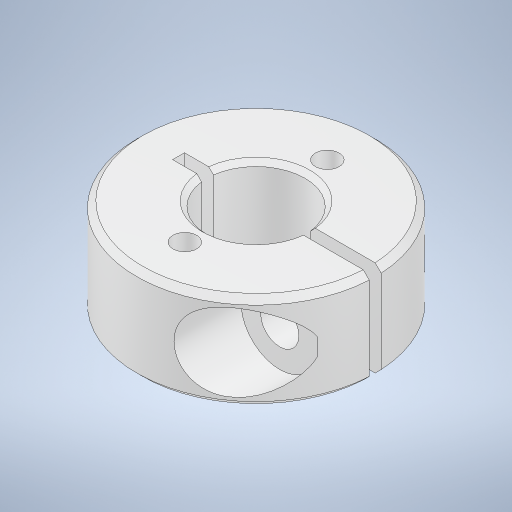
# Autodesk Inventor part: Collar
Saved by Autodesk Inventor 2023.4 (Build 274418000, 418)
## iProperties
Created: 2024-03-24
Part Number: Collar
Material: Aluminum 6061
Document SubType Name: Modeling
Designer: Nathan Cai
Density: 2.7 g/cm^3
Appearance: Aluminum - Flat
Author: Nathan Cai
Autodesk Inventor part; units mm, degrees
ref_plane "YZ Plane" through (0, 0, 0) normal (1, 0, 0) x (0, 1, 0)
ref_plane "XZ Plane" through (0, 0, 0) normal (0, 1, 0) x (-1, 0, 0)
sketch "Sketch1" plane through (0, 0, 0) normal (0, 1, 0) x (-1, 0, 0)
  circle A0 centre (0, 0) radius 4
  circle A1 centre (0, 0) radius 10
  dimension "d0" = 8
  dimension "d1" = 20
  constraints: 2 centre point, 2 coincident
  measures "d0" diameter of A0
  measures "d1" diameter of A1
extrude "Extrusion1" add sketch "Sketch1" along normal blind 8
chamfer "Chamfer1" distance 0.5 angle 45 4 edges at (4, 8, 0) (10, 8, 0) (10, 0, 0) (4, 0, 0)
thicken "Thicken1" operation add thickness 0.1 both sides no extend neighbours yes toward (-0.9967573, 0, -0.0804666) faces at (-3.987, 5.1667, -0.3219)
sketch "Sketch2" plane through (0, 8, 0) normal (0, 1, 0) x (1, 0, 0)
  circle A0 centre (0, 0) radius 4 construction
  line L0 (-4, 0) -> (0, 0) construction
  line L1 (9.9875, -0.5) -> (-6.5, -0.5)
  line L2 (-6.5, -0.5) -> (-6.5, 0.5)
  line L3 (-6.5, 0.5) -> (9.9875, 0.5)
  line L4 (9.9875, 0.5) -> (9.9875, -0.5) construction
  line L5 (9.9875, -0.5) -> (-6.5, 0.5) construction
  line L6 (-6.5, -0.5) -> (9.9875, 0.5) construction
  circle A1 centre (0, 0) radius 10 projected
  point P0 (1.7437, 0)
  dimension "d4" = 1
  dimension "d5" = 2.5
  constraints: 14 end point, 2 horizontal, 2 midpoint, 2 parallel, 1 horizontal alignment, 1 perpendicular, 1 point on line, 3 other
  measures "d4" distance of L1.end L2.end
  measures "d5" distance from line of L2 L0.start
extrude "Extrusion2" cut sketch "Sketch2" against normal through all contours L1 L2 L3 A1 picked at (-1, 0)
sketch "Sketch3" plane through (0, 0, 0) normal (0, -1, 0) x (1, 0, 0)
  circle A0 centre (0, 5.975) radius 1.875 construction
  arc A1 (4.0694, 0.5) -> (-4.0694, 0.5) centre (0, 0) ccw projected
  arc A2 (9.9875, 0.5) -> (9.9875, -0.5) centre (0, 0) ccw projected
  circle A3 centre (0, 5.975) radius 1
  line L0 (0, 0) -> (0, 10) construction
  line L1 (0, 0) -> (0, 5.975) construction
  circle A4 centre (0, -5.975) radius 1
  dimension "d11" = 3.75
  dimension "d12" = 2
  dimension "d15" = 0
  dimension "d18" = 360
  constraints: 4 end point, 3 centre point, 1 coincident, 1 point on circle, 1 tangent, 1 vertical, 5 other
  measures "d11" diameter of A0
  measures "d12" diameter of A3
  measures "d15" distance between parallel lines of L0 L1
extrude "Extrusion3" cut sketch "Sketch3" against normal through all
ref_plane "Work Plane1" through (0, 0, 7) normal (0, 0, 1) x (1, 0, 0)
sketch "Sketch4" plane through (0, 0, 7) normal (0, 0, 1) x (1, 0, 0)
  line L0 (-10, 0.5) -> (-10, 7.5) projected
  line L1 (-10, 4) -> (10, 4) construction
  line L2 (9.9875, 0.5) -> (9.9875, 7.5) projected
  point P0 (0, 0)
  point P1 (5.9875, 4)
  dimension "d21" = 4
  constraints: 2 end point, 1 horizontal, 1 midpoint, 1 point on line
  measures "d21" distance from line of L2 point (5.987, 4)
hole "Hole1" at (5.9875, 4, 7) direction (0, 0, -1) diameter 3.2004 end through all counterbore diameter 6.5024 counterbore depth 2.9972 clearance for "Socket Head Cap Screw" size "M3" standard "Ansi Metric M Profile"
delete faces "Delete Face1" heal yes whole lump no faces at (6.1413, 4.892, 7)
body "Solid1"
